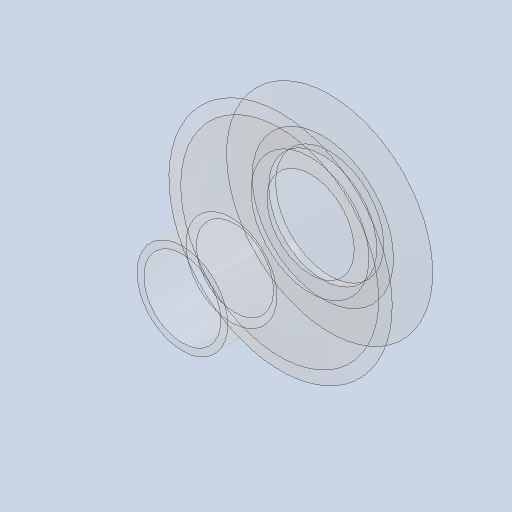
# Autodesk Inventor part: Ventosa
Saved by Autodesk Inventor 2023 (Build 270158000, 158)
## iProperties
Created: 2022-11-04
Part Number: Ventosa
Material: SAN Plastic
Document SubType Name: Modeling
Designer: Daniel Peña
Density: 1.068 g/cm^3
Appearance: Polycarbonate - Clear
Author: Daniel Peña
Autodesk Inventor part; units mm, degrees
ref_plane "YZ Plane" through (0, 0, 0) normal (1, 0, 0) x (0, 1, 0)
ref_plane "XZ Plane" through (0, 0, 0) normal (0, 1, 0) x (-1, 0, 0)
ref_plane "XY Plane" through (0, 0, 0) normal (0, 0, 1) x (1, 0, 0)
sketch "Sketch2" plane through (0, 0, 0) normal (1, 0, 0) x (0, 1, 0)
  line L0 (11, 0) -> (21, 0)
  line L1 (0, 0) -> (0, 40.0317)
  line L2 (21, 0) -> (12, 4)
  line L3 (12, 4) -> (22.75, 10)
  line L4 (22.75, 10) -> (9.25, 20)
  line L5 (9.25, 20) -> (9.25, 30)
  line L6 (9.25, 30) -> (7.85, 30)
  line L7 (7.85, 30) -> (7.85, 19.2948)
  line L8 (7.85, 19.2948) -> (20.1743, 10.1657)
  line L9 (20.1743, 10.1657) -> (8.8727, 3.8579)
  line L10 (8.8727, 3.8579) -> (14.4029, 1.4)
  line L11 (14.4029, 1.4) -> (11, 1.4)
  line L12 (11, 0) -> (11, 1.4)
  dimension "d10" = 22
  dimension "d11" = 42
  dimension "d12" = 24
  dimension "d13" = 4
  dimension "d14" = 10
  dimension "d15" = 45.5
  dimension "d16" = 18.5
  dimension "d17" = 10
  dimension "d18" = 10
  dimension "d19" = 1.4
  dimension "d20" = 1.4
  constraints: 26 end point, 3 vertical, 1 horizontal, 1 perpendicular, 1 point on line, 3 other
  measures "d10" diameter of L0.start L1
  measures "d11" diameter of L0.end L1
  measures "d12" diameter of L2.end L1
  measures "d13" vertical distance of L0.end L2.end
  measures "d14" distance from line of L0 L3.end
  measures "d15" diameter of L3.end L1
  measures "d16" diameter of L4.end L1
  measures "d17" vertical distance of L3.end L4.end
  measures "d18" distance of L4.end L5.end
  measures "d19" distance between parallel lines of L2 L10
  measures "d20" distance between parallel lines of L5 L7
revolve "Revolution1" add sketch "Sketch2" angle 360 about axis through (0, 0, 0) along (0, 0, 1)
body "Solid1"
